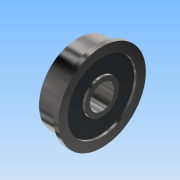
# Autodesk Inventor part: F625ZZ
Saved by Autodesk Inventor 2017 (Build 210142000, 142)
## iProperties
Part Number: F625ZZ
Material: Типовые
Document SubType Name: Modeling
Designer: Max
Mass: 0.841895 g
Surface Area: 8.72313 cm^2
Volume: 0.841895 cm^3
Density: 1 g/cm^3
Appearance: Сталь — полированная
Author: Max
Autodesk Inventor part; units mm, degrees
ref_plane "YZ Plane" through (0, 0, 0) normal (1, 0, 0) x (0, 1, 0)
ref_plane "XZ Plane" through (0, 0, 0) normal (0, 1, 0) x (-1, 0, 0)
ref_plane "XY Plane" through (0, 0, 0) normal (0, 0, 1) x (1, 0, 0)
sketch "Эскиз1" plane through (0, 0, 0) normal (1, 0, 0) x (0, 1, 0)
  circle A0 centre (0, 0) radius 8
  circle A1 centre (0, 0) radius 2.5
  circle A2 centre (0, 0) radius 9
  circle A3 centre (0, 0) radius 7.0758
  circle A4 centre (0, 0) radius 3.5071
  dimension "d0" = 16
  dimension "d1" = 5
  dimension "d2" = 18
  constraints: 5 centre point, 5 coincident
  measures "d0" diameter of A0
  measures "d1" diameter of A1
  measures "d2" diameter of A2
extrude "Выдавливание1" add sketch "Эскиз1" along normal mid plane 5 contours A0 | A4
extrude "Выдавливание2" add sketch "Эскиз1" along normal mid plane 4 contours A3
sketch "Эскиз2" plane through (2.5, 0, 0) normal (1, 0, 0) x (0, 0, -1)
  circle A0 centre (0, 0) radius 9
  circle A1 centre (0, 0) radius 8
  dimension "d7" = 18
  dimension "d8" = 16
  constraints: 2 centre point, 2 coincident
  measures "d7" diameter of A0
  measures "d8" diameter of A1
extrude "Выдавливание3" add sketch "Эскиз2" against normal blind 1
